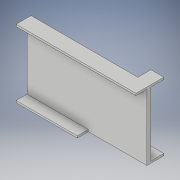
# Autodesk Inventor part: Guide
Saved by Autodesk Inventor 2019 (Build 230136000, 136)
## iProperties
Created: 2020-10-13
Part Number: Guide
Material: Generic
Document SubType Name: Modeling
Designer: Delta
Density: 1 g/cm^3
Appearance: Default
Author: Delta
Autodesk Inventor part; units mm, degrees
ref_plane "YZ Plane" through (0, 0, 0) normal (1, 0, 0) x (0, 1, 0)
ref_plane "XZ Plane" through (0, 0, 0) normal (0, 1, 0) x (-1, 0, 0)
ref_plane "XY Plane" through (0, 0, 0) normal (0, 0, 1) x (1, 0, 0)
sketch "Sketch1" plane through (0, 0, 0) normal (0, 0, 1) x (1, 0, 0)
  line L0 (0, 0) -> (233.68, 0)
  line L1 (233.68, 0) -> (233.68, 132.6642)
  line L2 (233.68, 132.6642) -> (0, 132.6642)
  line L3 (0, 132.6642) -> (0, 0)
  dimension "d0" = 132.6642
  dimension "d1" = 233.68
  constraints: 8 end point, 2 parallel, 1 horizontal, 1 perpendicular
  measures "d0" distance of L0.end L1.end
  measures "d1" distance of L1.end L2.end
extrude "Extrusion1" add sketch "Sketch1" along normal blind 29.21
sketch "Sketch2" plane through (0, 0, 29.21) normal (0, 0, 1) x (1, 0, 0)
  line L0 (-0.3825, 3.8354) -> (233.706, 3.8354)
  line L1 (233.706, 3.8354) -> (233.706, 128.8288)
  line L2 (233.706, 128.8288) -> (-0.3825, 128.8288)
  line L3 (-0.3825, 128.8288) -> (-0.3825, 3.8354)
  line L4 (233.68, 132.6642) -> (0, 132.6642) projected
  line L5 (0, 0) -> (233.68, 0) projected
  dimension "d4" = 3.8354
  dimension "d5" = 3.8354
  constraints: 8 end point, 2 parallel, 1 horizontal, 1 perpendicular
  measures "d4" distance between parallel lines of L4 L2
  measures "d5" distance between parallel lines of L5 L0
extrude "Extrusion2" cut sketch "Sketch2" against normal blind 21.4884
sketch "Sketch3" plane through (0, 0, 29.21) normal (0, 0, 1) x (1, 0, 0)
  line L0 (233.68, 0) -> (119.38, 0)
  line L1 (119.38, 0) -> (119.38, 3.8354)
  line L2 (119.38, 3.8354) -> (233.68, 3.8354)
  line L3 (233.68, 3.8354) -> (233.68, 0)
  point P0 (0, 0)
  dimension "d8" = 114.3
  dimension "d9" = 3.8354
  constraints: 8 end point, 2 parallel, 1 horizontal, 1 perpendicular
  measures "d8" distance of L1.end L2.end
  measures "d9" distance of L0.end L1.end
extrude "Extrusion3" cut sketch "Sketch3" against normal blind 21.4884
sketch "Sketch4" plane through (0, 0, 0) normal (0, 0, -1) x (-1, 0, 0)
  line L0 (-233.68, 0) -> (-233.68, 132.6642) projected
  line L1 (-233.68, 132.6642) -> (-208.28, 132.6642)
  line L2 (-208.28, 132.6642) -> (-208.28, 128.8288)
  line L3 (-208.28, 128.8288) -> (-233.68, 128.8288)
  line L4 (-233.68, 128.8288) -> (-233.68, 132.6642)
  line L5 (-233.68, 0) -> (-208.28, 0)
  line L6 (-208.28, 0) -> (-208.28, 3.8354)
  line L7 (-208.28, 3.8354) -> (-233.68, 3.8354)
  line L8 (-233.68, 3.8354) -> (-233.68, 0)
  point P0 (0, 0)
  dimension "d12" = 3.8354
  dimension "d13" = 25.4
  dimension "d14" = 3.8354
  dimension "d15" = 25.4
  constraints: 16 end point, 4 parallel, 2 horizontal, 2 perpendicular
  measures "d12" distance of L1.end L2.end
  measures "d13" distance of L2.end L3.end
  measures "d14" distance of L5.end L6.end
  measures "d15" distance of L6.end L7.end
extrude "Extrusion4" add sketch "Sketch4" along normal blind 25.4
body "Solid1"
